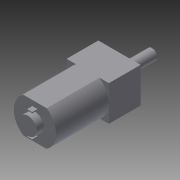
# Autodesk Inventor part: motor pololu
Saved by Autodesk Inventor 2013 (Build 170138000, 138)
## iProperties
Created: 2013-05-03
Part Number: motor pololu
Material: Generic
Document SubType Name: Modeling
Designer: otrab
Density: 1 g/cm^3
Author: otrab
Autodesk Inventor part; units mm, degrees
ref_plane "YZ Plane" through (0, 0, 0) normal (1, 0, 0) x (0, 1, 0)
ref_plane "XZ Plane" through (0, 0, 0) normal (0, 1, 0) x (-1, 0, 0)
ref_plane "XY Plane" through (0, 0, 0) normal (0, 0, 1) x (1, 0, 0)
sketch "Sketch1" plane through (0, 0, 0) normal (0, 1, 0) x (-1, 0, 0)
  line L0 (0, 0) -> (0, 5) construction
  line L1 (-3.3166, 5) -> (3.3166, 5)
  line L2 (-8.6998, 0) -> (12.7628, 0) construction
  line L3 (-3.3166, -5) -> (3.3166, -5)
  arc A0 (-3.3166, 5) -> (-3.3166, -5) centre (0, 0) ccw
  arc A1 (3.3166, -5) -> (3.3166, 5) centre (0, 0) ccw
  dimension "d1" = 5
  constraints: 8 end point, 4 point on circle, 2 centre point, 2 symmetric about line, 1 coincident, 1 parallel, 1 perpendicular, 1 vertical
  measures "d1" distance of L0.start L0.end
extrude "Extrusion1" add sketch "Sketch1" along normal blind 15
sketch "Sketch2" plane through (0, 15, 0) normal (0, 1, 0) x (1, 0, 0)
  arc A0 (-3.3166, 5) -> (-3.3166, -5) centre (0, 0) ccw projected
  line L0 (-6, -5) -> (6, -5)
  line L1 (6, -5) -> (6, 5)
  line L2 (6, 5) -> (-6, 5)
  line L3 (-6, 5) -> (-6, -5)
  line L4 (-6, -5) -> (6, 5) construction
  line L5 (6, -5) -> (-6, 5) construction
  constraints: 12 end point, 2 midpoint, 2 parallel, 1 horizontal, 1 perpendicular
extrude "Extrusion2" add sketch "Sketch2" along normal blind 9
sketch "Sketch3" plane through (0, 24, 0) normal (0, 1, 0) x (1, 0, 0)
  line L0 (-6, 5) -> (-6, -5) projected
  arc A0 (-1.118, 1) -> (1.118, 1) centre (0, 0) ccw
  line L1 (0, -1.5) -> (0, 1) construction
  line L2 (-1.118, 1) -> (1.118, 1)
  dimension "d6" = 3
  dimension "d7" = 2.5
  constraints: 4 end point, 3 point on circle, 1 centre point, 1 coincident, 1 parallel, 1 perpendicular
  measures "d6" diameter of A0
  measures "d7" distance of L1.start L1.end
extrude "Extrusion3" add sketch "Sketch3" along normal blind 9.27
sketch "Sketch5" plane through (0, 0, 0) normal (0, -1, 0) x (1, 0, 0)
  line L0 (0, 0) -> (0, 3.5) construction
  line L1 (0, 3.5) -> (0.75, 3.5)
  line L2 (0, 3.5) -> (-0.75, 3.5)
  line L3 (0.75, 3.5) -> (0.75, 3.2)
  line L4 (0.75, 3.2) -> (-0.75, 3.2)
  line L5 (-0.75, 3.2) -> (-0.75, 3.5)
  line L6 (7.0613, 0) -> (-6.7326, 0) construction
  line L7 (-0.75, -3.2) -> (-0.75, -3.5)
  line L8 (0.75, -3.2) -> (-0.75, -3.2)
  line L9 (0.75, -3.5) -> (0.75, -3.2)
  line L10 (0, 0) -> (0, -3.5) construction
  line L11 (0, -3.5) -> (0.75, -3.5)
  line L12 (0, -3.5) -> (-0.75, -3.5)
  dimension "d14" = 3.5
  dimension "d15" = 0.75
  dimension "d16" = 0.3
  constraints: 26 end point, 6 symmetric about line, 4 perpendicular, 1 parallel
  measures "d14" distance of L10.start L0.end
  measures "d15" distance of L0.end L1.end
  measures "d16" distance of L1.end L4.start
extrude "Extrusion4" add sketch "Sketch5" along normal blind 1.5
sketch "Sketch6" plane through (0, 0, 0) normal (0, -1, 0) x (1, 0, 0)
  arc A0 (3.3166, -5) -> (3.3166, 5) centre (0, 0) ccw projected
  circle A1 centre (0, 0) radius 2.5
  dimension "d19" = 5
  constraints: 1 centre point, 1 coincident
  measures "d19" diameter of A1
extrude "Extrusion5" add sketch "Sketch6" along normal blind 2
body "Solid1"
